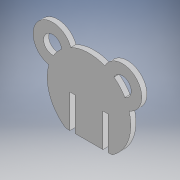
# Autodesk Inventor part: BackPiece
Saved by Autodesk Inventor 2019 (Build 230136000, 136)
## iProperties
Created: 2020-02-13
Part Number: BackPiece
Material: Generic
Document SubType Name: Modeling
Designer: student
Density: 1 g/cm^3
Appearance: Default
Author: student
Autodesk Inventor part; units mm, degrees
ref_plane "YZ Plane" through (0, 0, 0) normal (1, 0, 0) x (0, 1, 0)
ref_plane "XZ Plane" through (0, 0, 0) normal (0, 1, 0) x (-1, 0, 0)
ref_plane "XY Plane" through (0, 0, 0) normal (0, 0, 1) x (1, 0, 0)
sketch "Sketch1" plane through (0, 0, 0) normal (0, 0, 1) x (1, 0, 0)
  arc A0 (-16.5424, 34.3214) -> (-36.5756, 10.6694) centre (-33.2088, 28.1277) ccw
  arc A1 (36.5756, 10.6694) -> (16.5424, 34.3214) centre (33.2088, 28.1277) ccw
  arc A2 (-36.5756, 10.6694) -> (36.5756, 10.6694) centre (0, 0) ccw
  arc A3 (16.5424, 34.3214) -> (-16.5424, 34.3214) centre (0, 0) ccw
  dimension "d10" = 17.78
  dimension "d14" = 38.1
  dimension "d15" = 38.1
  dimension "d19" = 33.2088
  dimension "d20" = 33.2088
  dimension "d21" = 28.1277
  dimension "d22" = 28.1277
  constraints: 8 point on circle, 4 centre point, 1 coincident, 1 equal radius
  measures "d10" radius of A0
  measures "d14" radius of A2
  measures "d15" radius of A3
  measures "d19" horizontal distance of point (0, 0) A0.centre
  measures "d20" horizontal distance of point (0, 0) A1.centre
  measures "d21" vertical distance of point (0, 0) A0.centre
  measures "d22" vertical distance of point (0, 0) A1.centre
extrude "Extrusion1" add sketch "Sketch1" along normal blind 4.699
sketch "Sketch2" plane through (0, 0, 0) normal (0, 0, -1) x (-1, 0, 0)
  arc A0 (36.5756, 10.6694) -> (16.5424, 34.3214) centre (33.2088, 28.1277) ccw projected
  arc A1 (16.5424, 34.3214) -> (-16.5424, 34.3214) centre (0, 0) ccw projected
  arc A2 (-16.5424, 34.3214) -> (-36.5756, 10.6694) centre (-33.2088, 28.1277) ccw projected
  arc A3 (-36.5756, 10.6694) -> (36.5756, 10.6694) centre (0, 0) ccw projected
  arc A4 (-36.5756, 10.6694) -> (36.5756, 10.6694) centre (0, 0) ccw projected
  line L0 (-21.0606, -31.75) -> (21.0606, -31.75)
  point P0 (0, -38.1)
  dimension "d4" = 6.35
  constraints: 3 point on circle, 2 end point, 1 horizontal
  measures "d4" distance from line of L0 point (0, -38.1)
extrude "Extrusion2" cut sketch "Sketch2" against normal blind 25.4 contours A3 L0
fillet "Fillet1" radius 3.175 2 edges at (21.0606, -31.75, 2.3495) (-21.0606, -31.75, 2.3495)
sketch "Sketch3" plane through (0, 0, 4.699) normal (0, 0, 1) x (1, 0, 0)
  line L0 (-17.399, -1.27) -> (-12.7, -1.27) projected
  line L1 (20.0805, -31.75) -> (-20.0805, -31.75) projected
  line L2 (-17.399, -1.27) -> (-12.7, -1.27)
  line L3 (-12.7, -1.27) -> (-12.7, -31.75)
  line L4 (-12.7, -31.75) -> (-17.399, -31.75)
  line L5 (-17.399, -31.75) -> (-17.399, -1.27)
  point P0 (0, 0)
  constraints: 8 end point, 2 parallel, 1 horizontal, 1 perpendicular, 1 point on line
extrude "Extrusion3" cut sketch "Sketch3" against normal through all
mirror "Mirror1" about plane through (0, 0, 0) normal (1, 0, 0) of "Extrusion3"
sketch "Sketch5" plane through (0, 0, 4.699) normal (0, 0, 1) x (1, 0, 0)
  circle A0 centre (0, 0) radius 38.1
  arc A1 (16.5424, 34.3214) -> (-16.5424, 34.3214) centre (0, 0) ccw projected
  arc A2 (-25.0249, 28.7291) -> (-32.4554, 19.9564) centre (-33.2088, 28.1277) ccw
  arc A3 (-16.5424, 34.3214) -> (-36.5756, 10.6694) centre (-33.2088, 28.1277) ccw projected
  arc A4 (32.4554, 19.9564) -> (25.0249, 28.7291) centre (33.2088, 28.1277) ccw
  arc A5 (36.5756, 10.6694) -> (16.5424, 34.3214) centre (33.2088, 28.1277) ccw projected
  dimension "d16" = 10.16
  constraints: 8 point on circle, 3 centre point, 2 concentric, 2 equal radius, 1 coincident
  measures "d16" distance of A0.start A0.end
extrude "Extrusion5" cut sketch "Sketch5" against normal through all contours A0 A4 | A2 A0
equation "\"d20\" = d19"
equation "\"d22\" = d21"
body "Solid1"
